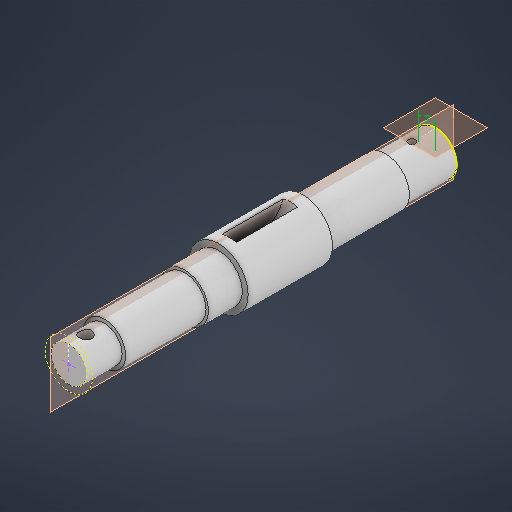
# Autodesk Inventor part: lab2_MarcuBianca
Saved by Autodesk Inventor 2026.2 (Build 302298010, 298A)
## iProperties
Created: 2026-03-02
Part Number: lab2_MarcuBianca
Material: Generic
Document SubType Name: Modeling
Designer: Bianca
Density: 1 g/cm^3
Appearance: Default
Author: Bianca
Autodesk Inventor part; units mm, degrees
ref_plane "XZ Plane" through (0, 0, 0) normal (0, 1, 0) x (-1, 0, 0)
ref_plane "XY Plane" through (0, 0, 0) normal (0, 0, 1) x (1, 0, 0)
sketch "Sketch1" plane through (0, 0, 0) normal (0, 1, 0) x (-1, 0, 0)
  line L0 (0, 112.724) -> (0, -42.276)
  line L1 (0, -42.276) -> (9, -42.276)
  line L2 (9, -42.276) -> (9, -21.276)
  line L3 (9, -21.276) -> (10, -21.276)
  line L4 (10, -21.276) -> (10, 13.724)
  line L5 (10, 13.724) -> (12.5, 13.724)
  line L6 (12.5, 13.724) -> (12.5, 49.424)
  line L7 (12.5, 49.424) -> (10, 49.424)
  line L8 (10, 49.424) -> (10, 63.724)
  line L9 (10, 63.724) -> (9, 63.724)
  line L10 (9, 63.724) -> (9, 97.724)
  line L11 (9, 97.724) -> (7.5, 97.724)
  line L12 (7.5, 97.724) -> (7.5, 112.724)
  line L13 (7.5, 112.724) -> (0, 112.724)
  point P0 (0, 0)
  dimension "d1" = 155
  dimension "d2" = 9
  dimension "d3" = 21
  dimension "d4" = 1
  dimension "d5" = 35
  dimension "d6" = 2.5
  dimension "d7" = 35.7
  dimension "d8" = 2.5
  dimension "d9" = 14.3
  dimension "d10" = 1
  dimension "d11" = 34
  dimension "d12" = 1.5
  dimension "d13" = 15
  dimension "d15" = 7.5
  constraints: 28 end point, 8 perpendicular, 2 point on line, 1 horizontal, 1 parallel, 1 vertical
  measures "d1" distance of L0.start L0.end
  measures "d2" distance of L0.end L1.end
  measures "d3" distance of L1.end L2.end
  measures "d4" distance of L2.end L3.end
  measures "d5" distance of L3.end L4.end
  measures "d6" distance of L4.end L5.end
  measures "d7" distance of L5.end L6.end
  measures "d8" distance of L6.end L7.end
  measures "d9" distance of L7.end L8.end
  measures "d10" distance of L8.end L9.end
  measures "d11" distance of L9.end L10.end
  measures "d12" distance of L10.end L11.end
  measures "d13" distance of L11.end L12.end
  measures "d15" distance of L12.end L0.start
revolve "Revolution1" add sketch "Sketch1" angle 360 about axis through (0, 0, 112.724) along (0, 0, -1)
sketch "Sketch2" plane through (0, 0, 112.724) normal (0, 0, 1) x (1, 0, 0)
  circle A0 centre (0, 0) radius 10 construction
  line L0 (0, 0) -> (0, 7.5) construction
  circle A1 centre (0, 0) radius 7.5 construction
  constraints: 6 coincident, 2 end point, 1 vertical, 1 vertical alignment, 1 other
ref_plane "Work Plane1" through (0, 7.5, 112.724) normal (0, 1, 0) x (-1, 0, 0)
sketch "Sketch3" plane through (0, 0, 112.724) normal (0, 0, 1) x (1, 0, 0)
  point P0 (0, 0)
sketch "Sketch5" plane through (0, 0, -42.276) normal (0, 0, -1) x (-1, 0, 0)
  point P0 (0, 0)
sketch "Sketch6" plane through (0, 0, -42.276) normal (0, 0, -1) x (-1, 0, 0)
  line L0 (0, 0) -> (0, 9)
  circle A0 centre (0, 0) radius 9 projected
  line L1 (0, 9) -> (0, 2.2312)
  line L2 (0, 0) -> (7, 0)
  dimension "d26" = 7
  constraints: 6 end point, 1 horizontal, 1 point on line, 1 vertical, 1 vertical alignment, 1 other
  measures "d26" distance of L2.start L2.end
ref_plane "Work Plane2" through (0, 9, -42.276) normal (0, 1, 0) x (-1, 0, 0)
sketch "Sketch7" plane through (0, 0, -42.276) normal (0, 0, -1) x (-1, 0, 0)
  point P0 (0, 0)
sketch "Sketch8" plane through (0, 9, -42.276) normal (0, 1, 0) x (-1, 0, 0)
  line L0 (-9, 0) -> (9, 0) projected
  line L1 (0, 0) -> (0, 10)
  circle A0 centre (0, 10) radius 2.5
  point P0 (0, 42.276)
  dimension "d27" = 10
  dimension "d28" = 5
  constraints: 2 end point, 1 centre point, 1 coincident, 1 midpoint, 1 vertical
  measures "d27" distance of L1.start L1.end
  measures "d28" diameter of A0
hole "Hole2" at (0, 9, -32.276) direction (0, -1, 0) diameter 3 end through all
sketch "Sketch9" plane through (0, 0, 13.724) normal (0, 0, -1) x (-1, 0, 0)
  point P0 (0, 0)
sketch "Sketch10" plane through (0, 0, 112.724) normal (0, 0, 1) x (1, 0, 0)
  point P0 (0, 0)
ref_plane "Work Plane3" through (0, 9, -42.276) normal (0, 1, 0) x (-1, 0, 0)
sketch "Sketch11" plane through (0, 0, -42.276) normal (0, 0, -1) x (-1, 0, 0)
  point P0 (0, 0)
sketch "Sketch12" plane through (0, 0, 0) normal (1, 0, 0) x (0, 1, 0)
  point P0 (0, 0)
sketch "Sketch13" plane through (0, 0, 0) normal (1, 0, 0) x (0, 1, 0)
  point P0 (0, 0)
sketch "Sketch14" plane through (0, 7.5, 112.724) normal (0, 1, 0) x (-1, 0, 0)
  point P0 (0, -112.724)
ref_plane "Work Plane6" through (0, 0, -42.276) normal (1, 0, 0) x (0, 1, 0)
sketch "Sketch15" plane through (0, 0, -42.276) normal (1, 0, 0) x (0, 1, 0)
  line L0 (-9, 140) -> (9, 140) projected
  line L1 (7.3106, 140) -> (-0.6894, 140)
  line L2 (7.5, 155) -> (7.5, 140) projected
  line L3 (7.5, 140) -> (7.5, 148)
  line L4 (7.5, 148) -> (7.5, 144.4296)
  line L5 (7.5, 148) -> (7.5, 145.35)
  line L6 (-7.5, 155) -> (-7.5, 140) projected
  line L7 (7.5, 148) -> (-7.5, 148)
  line L8 (-7.5, 146.2148) -> (-7.5, 148)
  line L9 (-7.5, 148) -> (-7.5, 145.5)
  line L10 (7.5, 148) -> (7.5, 145.35)
  line L11 (7.5, 145.35) -> (-7.711, 145.5)
  point P0 (0, 42.276)
  point P1 (-7.5, 145.4979)
  dimension "d36" = 8
  dimension "d38" = 8
  dimension "d41" = 2.5
  dimension "d42" = 2.65
  constraints: 18 end point, 8 point on line, 2 collinear, 1 perpendicular
  measures "d36" distance of L1.start L1.end
  measures "d38" distance of L2.end L3.end
  measures "d41" distance of L7.end L9.end
  measures "d42" distance of L3.end L5.end
sketch "Sketch16" plane through (0, 0, -42.276) normal (1, 0, 0) x (0, 1, 0)
  line L0 (12.5, 91.7) -> (12.5, 56) projected
  line L1 (12.5, 56) -> (12.5, 74)
  line L2 (12.5, 74) -> (26.6302, 74)
  line L3 (12.5, 74) -> (-12.5744, 74)
  line L4 (12.5, 74) -> (12.5, 91.3)
  line L5 (-12.5, 91.7) -> (12.5, 91.7) projected
  line L6 (0, 91.7) -> (17.3, 91.7)
  line L7 (17.3, 91.7) -> (17.3, 56.7834)
  arc A0 (12.4208, 87.196) -> (12.5, 61.2578) centre (17.3, 74.2417) ccw
  point P0 (0, 42.276)
  dimension "d43" = 18
  dimension "d46" = 17.3
  constraints: 12 end point, 4 point on line, 2 midpoint, 2 point on circle, 1 centre point, 1 collinear, 1 horizontal, 1 perpendicular
  measures "d43" distance of L1.start L1.end
  measures "d46" distance of L6.start L6.end
sketch "Sketch17" plane through (0, 0, -42.276) normal (1, 0, 0) x (0, 1, 0)
  point P0 (0, 42.276)
sketch "Sketch18" plane through (0, 0, -42.276) normal (1, 0, 0) x (0, 1, 0)
  point P0 (0, 42.276)
extrude "Extrusion1" cut sketch "Sketch16" along normal mid plane 6 fills toward (3.5074, 74.1996) open curves A0
sketch "Sketch19" plane through (0, 0, -42.276) normal (1, 0, 0) x (0, 1, 0)
  point P0 (0, 42.276)
revolve "Revolution2" cut sketch "Sketch15" angle 360 about axis through (0, 7.5, 105.724) along (0, 1, 0) contours L6 L7 L2 L11
body "Solid1"
